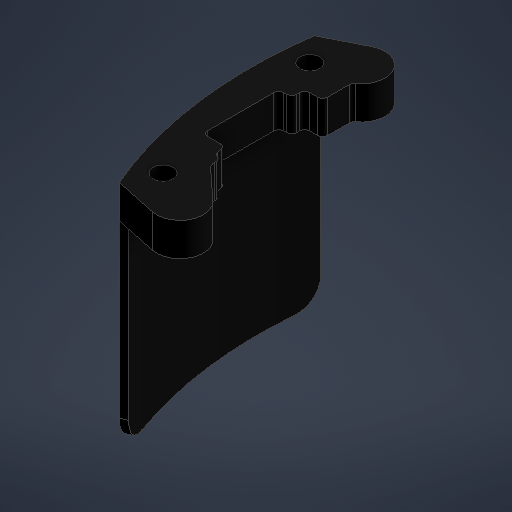
# Autodesk Inventor part: Abdeckung
Saved by Autodesk Inventor 2025.2 (Build 292293000, 293)
## iProperties
Created: 2025-03-12
Part Number: Abdeckung
Material: Generisch
Document SubType Name: Modeling
Designer: Faabs
Density: 1 g/cm^3
Appearance: Vorgabe
Author: Faabs
Autodesk Inventor part; units mm, degrees
ref_plane "YZ Plane" through (0, 0, 0) normal (1, 0, 0) x (0, 1, 0)
ref_plane "XZ Plane" through (0, 0, 0) normal (0, 1, 0) x (-1, 0, 0)
ref_plane "XY Plane" through (0, 0, 0) normal (0, 0, 1) x (1, 0, 0)
sketch "Skizze1" plane through (0, 0, 0) normal (0, 0, 1) x (1, 0, 0)
  circle A0 centre (0, 0) radius 88
  circle A1 centre (-82.6842, 7.2339) radius 2.1
  arc A2 (-78.002, 6.8243) -> (-73.5779, -26.7802) centre (0, 0) ccw
  circle A3 centre (-82.6842, 7.2339) radius 4.7
  circle A4 centre (-77.9945, -28.3877) radius 2.1
  circle A5 centre (-77.9945, -28.3877) radius 4.7
  circle A6 centre (0, 0) radius 78.3
  circle A7 centre (0, 0) radius 86.5
  arc A8 (-84.1729, 21.9984) -> (-86.4353, 9.8964) centre (0, 0) ccw
  line L0 (0, 0) -> (-82.0101, 11.8853)
  line L1 (-82.0101, 11.8853) -> (-87.0902, 12.6216)
  line L2 (0, 0) -> (-76.1395, -32.7061)
  line L3 (-76.1395, -32.7061) -> (-80.8559, -34.7321)
  line L4 (0, 0) -> (-82.828, 2.5361)
  line L5 (-82.828, 2.5361) -> (-87.9588, 2.6932)
  line L6 (0, 0) -> (-79.3493, -23.8872)
  line L7 (-79.3493, -23.8872) -> (-84.2646, -25.3669)
  line L8 (-78.3816, 80.7625) -> (-42.1157, 57.6586)
  line L9 (-42.1157, 57.6586) -> (-70.0553, 13.8022)
  line L10 (-70.0553, 13.8022) -> (-106.3212, 36.9061)
  line L11 (-106.3212, 36.9061) -> (-78.3816, 80.7625)
  line L12 (-56.0855, 35.7304) -> (-92.3514, 58.8343) construction
  line L13 (-64.096, -31.4636) -> (-25.7575, -66.5943)
  line L14 (-25.7575, -66.5943) -> (-54.8079, -98.2972)
  line L15 (-54.8079, -98.2972) -> (-93.1463, -63.1665)
  line L16 (-93.1463, -63.1665) -> (-64.096, -31.4636)
  line L17 (-47.7296, -52.0877) -> (-73.9771, -80.7319) construction
  arc A9 (-44.3621, 76) -> (44.3621, 76) centre (0, 0) ccw
  line L18 (13, 63) -> (-13, 63)
  line L19 (0, 63) -> (0, -88)
  line L20 (0, 0) -> (-56.0855, 35.7304) construction
  line L21 (0, 0) -> (-44.9267, -49.0289) construction
  line L22 (0, 0) -> (-88, 0)
  line L23 (0, 0) -> (-86.6631, 15.281) construction
  line L24 (0, 0) -> (-79.7551, -37.1904) construction
  circle A10 centre (0, 0) radius 83 construction
  line L25 (-63.2545, -17.7499) -> (-72.5045, -17.7499)
  arc A11 (-72.5045, -17.7499) -> (-74.5045, -19.7499) centre (-72.5045, -19.7499) ccw
  line L26 (-74.5045, -19.7499) -> (-74.5045, -21.0458)
  arc A12 (-74.5045, -21.0458) -> (-73.8556, -22.5204) centre (-72.5045, -21.0458) ccw
  line L27 (-73.8556, -22.5204) -> (-71.5045, -24.6748)
  line L28 (-71.5045, -24.6748) -> (-52.6253, -41.9744)
  arc A13 (-52.6253, -41.9744) -> (-51.2741, -42.4999) centre (-51.2741, -40.4999) ccw
  line L29 (-51.2741, -42.4999) -> (51.2741, -42.4999)
  arc A14 (51.2741, -42.4999) -> (52.6253, -41.9744) centre (51.2741, -40.4999) ccw
  line L30 (52.6253, -41.9744) -> (71.5045, -24.6748)
  line L31 (71.5045, -24.6748) -> (73.8557, -22.5204)
  arc A15 (73.8557, -22.5204) -> (74.5045, -21.0458) centre (72.5045, -21.0458) ccw
  line L32 (74.5045, -21.0458) -> (74.5045, -19.7499)
  arc A16 (74.5045, -19.7499) -> (72.5045, -17.7499) centre (72.5045, -19.7499) ccw
  line L33 (72.5045, -17.7499) -> (63.2545, -17.7499)
  arc A17 (61.2545, -15.7499) -> (63.2545, -17.7499) centre (63.2545, -15.7499) ccw
  line L34 (61.2545, -15.7499) -> (61.2545, -2.2499)
  arc A18 (63.2545, -0.2499) -> (61.2545, -2.2499) centre (63.2545, -2.2499) ccw
  line L35 (63.2545, -0.2499) -> (72.5045, -0.2499)
  arc A19 (72.5045, -0.2499) -> (74.5045, 1.7501) centre (72.5045, 1.7501) ccw
  line L36 (74.5045, 1.7501) -> (74.5045, 6.2357)
  arc A20 (74.5045, 6.2357) -> (74.1913, 7.3103) centre (72.5045, 6.2357) ccw
  line L37 (74.1913, 7.3103) -> (66.8685, 18.8046)
  line L38 (66.8685, 18.8046) -> (66.8312, 18.8625)
  line L39 (66.8312, 18.8625) -> (63.3633, 24.3061)
  line L40 (63.3633, 24.3061) -> (61.5013, 27.2292)
  arc A21 (61.5013, 27.2292) -> (61.4647, 27.2866) centre (58.5872, 25.413) ccw
  line L41 (61.4647, 27.2866) -> (59.6025, 30.21)
  line L42 (59.6025, 30.21) -> (59.5849, 30.2372)
  line L43 (59.5849, 30.2372) -> (52.3622, 41.5747)
  arc A22 (52.3622, 41.5747) -> (50.6754, 42.5001) centre (50.6754, 40.5001) ccw
  line L44 (50.6754, 42.5001) -> (34.4476, 42.5001)
  arc A23 (33.1728, 42.9591) -> (34.4476, 42.5001) centre (34.4477, 44.5002) ccw
  arc A24 (33.1728, 42.9591) -> (28.0733, 42.9591) centre (30.623, 39.877) ccw
  arc A25 (26.7984, 42.5001) -> (28.0733, 42.9591) centre (26.7984, 44.5002) ccw
  line L45 (26.7984, 42.5001) -> (-26.7984, 42.5001)
  arc A26 (-28.0733, 42.9591) -> (-26.7984, 42.5001) centre (-26.7984, 44.5002) ccw
  arc A27 (-28.0733, 42.9591) -> (-33.1728, 42.9591) centre (-30.623, 39.877) ccw
  arc A28 (-34.4476, 42.5001) -> (-33.1728, 42.9591) centre (-34.4477, 44.5002) ccw
  line L46 (-34.4476, 42.5001) -> (-50.6754, 42.5001)
  arc A29 (-50.6754, 42.5001) -> (-52.3622, 41.5747) centre (-50.6754, 40.5001) ccw
  line L47 (-52.3622, 41.5747) -> (-59.5849, 30.2372)
  line L48 (-59.5849, 30.2372) -> (-59.6025, 30.21)
  line L49 (-59.6025, 30.21) -> (-61.4647, 27.2866)
  arc A30 (-61.4647, 27.2866) -> (-61.5013, 27.2292) centre (-58.5191, 25.37) ccw
  line L50 (-61.5013, 27.2292) -> (-63.3633, 24.3061)
  line L51 (-63.3633, 24.3061) -> (-66.8312, 18.8625)
  line L52 (-66.8312, 18.8625) -> (-66.8685, 18.8046)
  line L53 (-66.8685, 18.8046) -> (-74.1912, 7.3103)
  arc A31 (-74.1912, 7.3103) -> (-74.5045, 6.2357) centre (-72.5045, 6.2357) ccw
  line L54 (-74.5045, 6.2357) -> (-74.5045, 1.7501)
  arc A32 (-74.5045, 1.7501) -> (-72.5045, -0.2499) centre (-72.5045, 1.7501) ccw
  line L55 (-72.5045, -0.2499) -> (-63.2545, -0.2499)
  arc A33 (-61.2545, -2.2499) -> (-63.2545, -0.2499) centre (-63.2545, -2.2499) ccw
  line L56 (-61.2545, -2.2499) -> (-61.2545, -15.7499)
  arc A34 (-63.2545, -17.7499) -> (-61.2545, -15.7499) centre (-63.2545, -15.7499) ccw
  line L57 (-82.6842, 7.2339) -> (-80.4481, 20.4232)
  circle A35 centre (-76.8409, 12.298) radius 4.9146
  circle A36 centre (-76.8409, 12.298) radius 4
  line L58 (-74.5045, 1.7501) -> (-78.2804, 1.7501)
  line L59 (-74.5045, -19.7499) -> (-75.7683, -19.7499)
  line L60 (-87.0902, 12.6216) -> (-79.059, 16.6835)
  line L61 (-77.9945, -28.3877) -> (-72.421, -40.5488)
  circle A37 centre (-71.0396, -31.7667) radius 4.9146
  circle A38 centre (-71.0396, -31.7667) radius 4
  line L62 (-80.8559, -34.7321) -> (-72.0471, -36.577)
  line L63 (-74.5045, 6.2357) -> (-74.5045, 10.7976)
  line L64 (-77.9945, -28.3877) -> (-73.2945, -28.3877)
  line L65 (-73.2945, -28.3877) -> (-73.2945, -31.484)
  line L66 (-73.2945, -28.3877) -> (-73.2945, -23.0346)
  point P0 (0, 0)
  point P1 (-85.6057, 12.4064)
  point P2 (-79.4777, -34.1401)
  point P3 (0, 0)
  point P4 (-74.9054, -43.26)
  point P5 (-83.5496, 22.399)
  point P6 (-86.1005, 12.4781)
  point P7 (-86.4122, 10.096)
  point P8 (-71.9434, -30.9037)
  point P9 (-77.4904, 11.2303)
  point P10 (-72.696, 9.6574)
  point P11 (-67.7194, -28.1432)
  point P12 (-67.103, -28.8245)
  point P13 (-74.5045, 7.9743)
  dimension "d0" = 9.4
  dimension "d1" = 173
  dimension "d8" = 52
  dimension "d9" = 43
  dimension "d10" = 43
  dimension "d11" = 52
  dimension "d12" = 66.5
  dimension "d13" = 90
  dimension "d14" = 90
  dimension "d15" = 90
  dimension "d16" = 90
  dimension "d17" = 90
  dimension "d18" = 90
  dimension "d19" = 90
  dimension "d20" = 66.5
  dimension "d21" = 26
  dimension "d22" = 47.5
  dimension "d23" = 32.5
  dimension "d139" = 10
  dimension "d140" = 25
  dimension "d156" = 8
  dimension "d157" = 8
  constraints: 134 end point, 73 point on circle, 37 centre point, 10 coincident, 10 point on line, 5 midpoint, 5 perpendicular, 5 tangent, 3 horizontal, 3 parallel, 2 vertical, 1 concentric, 16 other
  measures "d0" diameter of A5
  measures "d1" diameter of A7
  measures "d8" distance of L10.end L8.start
  measures "d9" distance of L9.end L10.end
  measures "d10" distance of L15.end L13.start
  measures "d11" distance of L14.end L15.end
  measures "d12" distance from line of L9 L20.start
  measures "d13" angle of L9 L20
  measures "d14" angle of L12 L9
  measures "d15" angle of L8 L9
  measures "d16" angle of L14 L13
  measures "d17" angle of L16 L13
  measures "d18" angle of L13 L17
  measures "d19" angle of L13 L21
  measures "d20" distance of L20.start L21.end
  measures "d21" distance between parallel lines of L20 L8
  measures "d22" angle of L22 L21
  measures "d23" angle of L22 L20
  measures "d139" angle of L22 L23
  measures "d140" angle of L24 L22
  measures "d156" diameter of A36
  measures "d157" diameter of A38
extrude "Extrusion1" add sketch "Skizze1" against normal blind 41 contours A0 L7 A7 A5 L3 | L1 A8 A3 A7 L5 A0 | A0 L22 A7 L7 | L5 A7 L22 A0 | L1 A7 A3 A8 | A5 A7 | A3 A7
extrude "Extrusion2" add sketch "Skizze1" along normal blind 7 contours A0 L7 A7 A5 L3 | L3 A7 L62 | L1 A8 A3 A7 L5 A0 | L60 A8 L1 | A0 L22 A7 L7 | L3 A5 L61 L62 A7 | A7 A5 L3 | L5 A7 L22 A0 | L1 A7 A3 A8 | A8 L60 A7 L1 | L60 L57 A3 L1 A7 | L7 A5 A7 | A7 L22 A2 L6 L7 | A7 A5 A37 L64 A4 L61 | A5 A7 | L61 A37 L62 | A37 L2 A38 A6 | A6 A38 L2 A37 | L54 L58 A2 L4 | L4 A2 A6 A35 L63 L54 | A12 L27 L66 A37 A6 A2 L6 | L6 A2 L59 L26 A12 | L5 L4 A2 L22 A7 | A7 A3 L5 | A3 A7 | L1 A3 A7 | L60 A35 L57 | A35 L0 A36 A6 | A6 A36 L0 A35 | L6 A2 A5 | L61 A4 L64 A37 A5 | A5 A37 L2 | L2 A37 L61 | A38 L2 A6 | A6 L2 A38 | A35 L63 A36 L0 | L2 A38 A6 L66 A37 | A37 L66 L27 L28 | L4 A3 A2 | A7 A3 A35 | A35 L0 L57 | A36 L0 A6 | A6 L0 A36 | A6 A37 A5 | A37 L64 A5 A38 | A5 A38 L2 A37 | L2 L65 A38 A6 | A6 A38 L2 | A38 A5 L65 L2 | A36 L63 L0 | A35 A6 A36 L63 | L66 A6 A37 | A3 A35 A6 | L0 A35 A3 | L0 A36 A3 A35 | L0 L63 A36 A6 | A6 A36 A3 L0 | A37 A6 L66 A5 | A5 L64 A37 | A38 A5 | A38 A5 L66 A6 | A35 A3 A36 A6 | A3 A36 A35 | A3 A36
sketch "Skizze7" plane through (0, 0, 7) normal (0, 0, 1) x (1, 0, 0)
  arc A0 (-75.2406, -20.5635) -> (-69.3003, -22.9246) centre (-71.3821, -19.509) ccw
  arc A1 (-77.999, 0.3892) -> (-75.2406, -20.5635) centre (0, 0) ccw
  arc A2 (-72.8723, 4.2072) -> (-77.999, 0.3892) centre (-73.9991, 0.3692) ccw
  arc A3 (-72.8723, 4.2072) -> (-61.6214, 8.4293) centre (-70.0553, 13.8022) ccw
  arc A4 (-73.0131, 3.7275) -> (-61.1997, 8.1606) centre (-70.0553, 13.8022) ccw
  arc A5 (-73.0131, 3.7275) -> (-77.499, 0.3867) centre (-73.9991, 0.3692) ccw
  arc A6 (-77.499, 0.3867) -> (-74.7582, -20.4317) centre (0, 0) ccw
  arc A7 (-74.7582, -20.4317) -> (-69.5605, -22.4976) centre (-71.3821, -19.509) ccw
  arc A8 (-57.0023, -23.7222) -> (-69.5605, -22.4976) centre (-64.096, -31.4636) ccw
  line L0 (-81.0045, -17) -> (-62.0045, -17)
  line L1 (-62.0045, -17) -> (-62.0045, -1)
  line L2 (-62.0045, -1) -> (-81.0045, -1)
  line L3 (-81.0045, -1) -> (-81.0045, -17)
  line L4 (-81.0045, -17) -> (-62.0045, -1) construction
  line L5 (-62.0045, -17) -> (-81.0045, -1) construction
  arc A9 (-75.2406, -20.5635) -> (-69.3003, -22.9246) centre (-71.3821, -19.509) ccw
  arc A10 (-77.999, 0.3892) -> (-75.2406, -20.5635) centre (0, 0) ccw
  arc A11 (-72.8723, 4.2072) -> (-77.999, 0.3892) centre (-73.9991, 0.3692) ccw
  arc A12 (-72.8723, 4.2072) -> (-61.6214, 8.4293) centre (-70.0553, 13.8022) ccw
  arc A13 (-73.0131, 3.7275) -> (-61.1997, 8.1606) centre (-70.0553, 13.8022) ccw
  arc A14 (-73.0131, 3.7275) -> (-77.499, 0.3867) centre (-73.9991, 0.3692) ccw
  arc A15 (-77.499, 0.3867) -> (-74.7582, -20.4317) centre (0, 0) ccw
  arc A16 (-74.7582, -20.4317) -> (-69.5605, -22.4976) centre (-71.3821, -19.509) ccw
  arc A17 (-57.0023, -23.7222) -> (-69.5605, -22.4976) centre (-64.096, -31.4636) ccw
  line L6 (0, 0) -> (-88, 0) construction
  line L7 (0, 0) -> (-70.4769, -25.6515) construction
  line L8 (0, 0) -> (-74.7146, 6.5367) construction
  circle A18 centre (-74.7146, 6.5367) radius 3
  line L9 (-74.7146, 6.5367) -> (-74.7146, -9.8771) construction
  line L10 (-78.7146, 6.5367) -> (-78.7146, -9.8771)
  line L11 (-70.7146, -9.8771) -> (-70.7146, 6.5367)
  arc A19 (-78.7146, -9.8771) -> (-70.7146, -9.8771) centre (-74.7146, -9.8771) ccw
  line L12 (-70.4769, -25.6515) -> (-70.4769, -13.0481) construction
  line L13 (-66.4769, -25.6515) -> (-66.4769, -13.0481)
  line L14 (-74.4769, -13.0481) -> (-74.4769, -25.6515)
  arc A20 (-66.4769, -13.0481) -> (-74.4769, -13.0481) centre (-70.4769, -13.0481) ccw
  point P0 (83.6944, 461.4718)
  point P1 (50.4138, 461.4718)
  point P2 (51.6944, 461.4718)
  point P3 (82.4138, 461.4718)
  point P4 (225.0044, 602.8331)
  point P5 (191.7237, 602.8331)
  point P6 (193.0044, 602.8331)
  point P7 (223.7237, 602.8331)
  point P8 (363.5869, 628.2091)
  point P9 (357.6097, 628.732)
  point P10 (362.0169, 595.2563)
  point P11 (367.655, 597.3084)
  point P12 (406.3129, 669.9339)
  point P13 (410.3051, 673.6839)
  point P14 (281.6601, 684.5107)
  point P15 (276.0219, 682.4586)
  point P16 (276.7768, 680.2764)
  point P17 (229.3797, 602.3331)
  point P18 (240.8641, 609.8331)
  point P19 (280.2544, 653.8611)
  point P20 (280.0901, 651.5579)
  point P21 (286.0672, 651.035)
  point P22 (286.3631, 657.444)
  point P23 (283.6046, 678.3966)
  point P24 (208.3641, 735.8331)
  point P25 (208.3641, 713.8331)
  point P26 (208.3641, 669.8331)
  point P27 (208.3641, 666.8331)
  point P28 (208.3641, 602.3331)
  point P29 (-74.7146, -1.6702)
  point P30 (-70.4769, -19.3498)
  point P31 (-61.892, 765.0568)
  point P32 (-53.892, 765.0568)
  point P33 (-66.1297, 787.0568)
  point P34 (-58.1297, 787.0568)
  point P35 (280.1559, 614.5868)
  point P36 (280.8975, 610.8357)
  point P37 (282.7456, 598.5868)
  dimension "d88" = 19
  dimension "d89" = 16
  dimension "d106" = 8
  dimension "d107" = 8
  constraints: 40 point on circle, 34 end point, 21 centre point, 5 parallel, 4 tangent, 3 coincident, 2 midpoint, 1 perpendicular, 6 other
  measures "d88" distance of L2.end L1.end
  measures "d89" distance of L1.end L0.end
  measures "d106" diameter of A19
  measures "d107" diameter of A20
extrude "Extrusion6" cut sketch "Skizze7" against normal blind 41 contours L0 L3 L2 L10 A19 A1 | A1 A19 A6 L0 | A19 L10 L2 A1 | A1 L2 A6 A19 | A6 A19 L14 L0 | L14 A19 L11 A20 L13 L0 | A6 L2 L11 A20 L14 A19 | L13 A20 L11 L2 L1 L0 | L14 A20 L11 A19
fillet "Rundung2" radius 1 9 edges at (-81.0045, -17, 3.5) (-81.0045, -1, 3.5) (-78.2936, -1, 3.5) (-78.2804, 1.7501, 3.5) (-74.5045, 1.7501, 3.5) (-76.4323, -17, 3.5) (-75.7683, -19.7499, 3.5) (-74.5045, -19.7499, 3.5) (-74.5045, 7.9743, 3.5)
fillet "Rundung3" radius 5 2 edges at (-86.3479, 12.514, -41) (-80.1668, -34.4361, -41)
equation "\"d10\" = d9"
equation "\"d11\" = d8"
